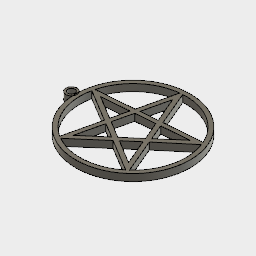
挂件1 v91 (Autodesk Fusion 360 design; units mm, degrees)
Autodesk Fusion 360 part; units mm, degrees
sketch "草图1" plane through (0, 0, 0) normal (0, 1, 0) x (1, 0, 0)
  line L0 (-14.2935, -6.0254) -> (-20.2817, -31.6727)
  circle A0 centre (0, 0) radius 40.6099
  line L1 (-2.6169, 30.7907) -> (-7.0044, 11.9991)
  line L2 (-4.1593, 37.3792) -> (-10.1475, 11.732)
  line L3 (-10.8647, 8.6602) -> (-13.5763, -2.9537)
  line L4 (-2.6169, 30.7907) -> (4.879, 13.0091)
  line L5 (-2.2085, 37.545) -> (8.022, 13.2762)
  line L6 (9.2473, 10.3695) -> (13.88, -0.6202)
  line L7 (15.1053, -3.5268) -> (25.3359, -27.7956)
  line L8 (6.1043, 10.1024) -> (11.4943, -2.6837)
  line L9 (12.7196, -5.5904) -> (20.2154, -23.372)
  line L10 (9.2473, 10.3695) -> (28.475, 12.0037)
  line L11 (8.022, 13.2762) -> (34.2645, 15.5065)
  line L12 (-30.0924, 7.026) -> (-13.5763, -2.9537)
  line L13 (-30.0924, 7.026) -> (-10.8647, 8.6602)
  line L14 (-7.7216, 8.9273) -> (6.1043, 10.1024)
  line L15 (-36.3899, 9.5016) -> (-10.1475, 11.732)
  line L16 (-7.0044, 11.9991) -> (4.879, 13.0091)
  line L17 (-36.835, 7.5951) -> (-14.2935, -6.0254)
  line L18 (-7.7216, 8.9273) -> (-10.8765, -4.585)
  line L19 (-11.5937, -7.6568) -> (-15.9812, -26.4484)
  line L20 (-15.9812, -26.4484) -> (-1.3862, -13.8246)
  line L21 (-10.8765, -4.585) -> (0.9996, -11.761)
  line L22 (3.6994, -13.3923) -> (20.2154, -23.372)
  line L23 (-18.606, -32.6852) -> (1.3136, -15.4559)
  line L24 (3.6994, -13.3923) -> (12.7196, -5.5904)
  line L25 (-11.5937, -7.6568) -> (-1.3862, -13.8246)
  line L26 (1.3136, -15.4559) -> (23.8551, -29.0764)
  line L27 (0.9996, -11.761) -> (11.4943, -2.6837)
  line L28 (13.88, -0.6202) -> (28.475, 12.0037)
  line L29 (15.1053, -3.5268) -> (35.1801, 13.2991)
  arc A1 (34.2645, 15.5065) -> (-2.2085, 37.545) centre (0, 0) ccw
  arc A2 (-4.1593, 37.3792) -> (-36.3899, 9.5016) centre (0, 0) ccw
  arc A3 (-36.835, 7.5951) -> (-20.2817, -31.6727) centre (0, 0) ccw
  arc A4 (-18.606, -32.6852) -> (23.8551, -29.0764) centre (0, 0) ccw
  arc A5 (25.3359, -27.7956) -> (35.1801, 13.2991) centre (0, 0) ccw
extrude "拉伸1" add sketch "草图1" along normal blind 5 makes body 1
sketch "草图2" plane through (0, 0, 0) normal (0, 1, 0) x (1, 0, 0)
  circle A0 centre (-55, 0) radius 2.5
  circle A1 centre (-55, 0) radius 4
  dimension "d6" = 5
  dimension "d7" = 8
  measures "d6" diameter of A0
  measures "d7" diameter of A1
extrude "拉伸2" add sketch "草图2" along normal blind 5 separate body makes body 2
move_body "移动1" bodies 2 to x (1, 0, 0) y (0, 1, 0) z (0, 0, 1) at (11.3, 0, 0)
